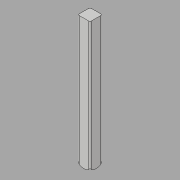
# Autodesk Inventor part: One_sided_axle_base-40_nogroove
Saved by Autodesk Inventor 2020 (Build 240168000, 168)
## iProperties
Created: 2018-11-05
Part Number: One_sided_axle_base-40_nogroove
Material: Generic
Description: Unknown
Document SubType Name: Modeling
Designer: Varga Daniel
Density: 1 g/cm^3
Appearance: Default
Company: Unknown
Sending System: DEX
Preprocessor: ST-DEVELOPER v16.7
Axle_length: 40,000 mm
Upper_fillet: 0,400 mm
Title: Axeis 2
Author: Unknown
Autodesk Inventor part; units mm, degrees
ref_plane "XZ Plane" through (0, 0, 0) normal (0, 1, 0) x (-1, 0, 0)
derived "Base_part.ipt"
sketch "Axle_sketch" plane through (0, 0, 0) normal (0, 1, 0) x (-1, 0, 0)
  circle A0 centre (0, 0) radius 2.5 construction
  line L0 (1.475, -1.875) -> (-1.475, -1.875)
  line L1 (-1.875, -1.475) -> (-1.875, 1.475)
  line L2 (-1.475, 1.875) -> (1.475, 1.875)
  line L3 (1.875, 1.475) -> (1.875, -1.475)
  line L4 (1.875, -1.875) -> (-1.875, 1.875) construction
  line L5 (-1.875, -1.875) -> (1.875, 1.875) construction
  arc A1 (1.475, -1.875) -> (1.875, -1.475) centre (1.475, -1.475) ccw
  arc A2 (-1.875, -1.475) -> (-1.475, -1.875) centre (-1.475, -1.475) ccw
  arc A3 (1.875, 1.475) -> (1.475, 1.875) centre (1.475, 1.475) ccw
  arc A4 (-1.475, 1.875) -> (-1.875, 1.475) centre (-1.475, 1.475) ccw
sketch "Sketch1" plane through (0, 0, 0) normal (0, 1, 0) x (-1, 0, 0)
  line L0 (-1.475, -1.875) -> (1.475, -1.875)
  line L1 (1.875, -1.475) -> (1.875, 1.475)
  line L2 (1.475, 1.875) -> (-1.475, 1.875)
  line L3 (-1.875, 1.475) -> (-1.875, -1.475)
  line L4 (-1.875, -1.875) -> (1.875, 1.875) construction
  line L5 (1.875, -1.875) -> (-1.875, 1.875) construction
  arc A0 (-1.875, -1.475) -> (-1.475, -1.875) centre (-1.475, -1.475) ccw
  arc A1 (1.475, -1.875) -> (1.875, -1.475) centre (1.475, -1.475) ccw
  arc A2 (1.875, 1.475) -> (1.475, 1.875) centre (1.475, 1.475) ccw
  arc A3 (-1.475, 1.875) -> (-1.875, 1.475) centre (-1.475, 1.475) ccw
  circle A4 centre (0, 0) radius 2.5 construction
  line L6 (1.475, -1.875) -> (-1.475, -1.875) construction
  arc A5 (1.475, -1.875) -> (1.875, -1.475) centre (1.475, -1.475) ccw construction
  line L7 (1.875, 1.475) -> (1.875, -1.475) construction
  circle A6 centre (0, 0) radius 2.5 construction
  line L8 (-1.475, 1.875) -> (1.475, 1.875) construction
  arc A7 (-1.475, 1.875) -> (-1.875, 1.475) centre (-1.475, 1.475) ccw construction
  line L9 (-1.875, -1.475) -> (-1.875, 1.475) construction
  arc A8 (-1.875, -1.475) -> (-1.475, -1.875) centre (-1.475, -1.475) ccw construction
  arc A9 (1.875, 1.475) -> (1.475, 1.875) centre (1.475, 1.475) ccw construction
  line L10 (-1.875, 1.875) -> (1.875, 1.875)
  line L11 (1.875, 1.875) -> (1.875, -1.875)
  line L12 (1.875, -1.875) -> (-1.875, -1.875)
  line L13 (-1.875, -1.875) -> (-1.875, 1.875)
  line L14 (1.875, -0.5) -> (0.875, -0.5)
  line L15 (0.875, -0.5) -> (0.875, 0.5)
  line L16 (0.875, 0.5) -> (1.875, 0.5)
  line L17 (1.875, 0.5) -> (1.875, -0.5)
  line L18 (-1.875, -0.5) -> (-0.875, -0.5)
  line L19 (-0.875, -0.5) -> (-0.875, 0.5)
  line L20 (-0.875, 0.5) -> (-1.875, 0.5)
  line L21 (-1.875, 0.5) -> (-1.875, -0.5)
  line L22 (-1.875, 0) -> (1.875, 0) construction
  point P0 (1.875, 1.475)
  point P1 (1.475, -1.875)
  point P2 (-1.875, -1.475)
  dimension "d0" = 3.75
  dimension "d1" = 3.75
  dimension "d2" = 0.4
  dimension "d11" = 5
  dimension "d13" = 3.75
  dimension "d14" = 0.4
  dimension "d31" = 1
  dimension "d32" = 1
  dimension "d33" = 1
  constraints: 38 end point, 12 point on line, 8 parallel, 8 point on circle, 8 tangent, 5 centre point, 5 midpoint, 4 collinear, 4 horizontal, 4 perpendicular, 3 equal radius, 1 coincident
  measures "d0" distance of L4.end L5.end
  measures "d1" distance between parallel lines of L2 L0
  measures "d2" radius of A0
  measures "d11" diameter of A4
  measures "d13" distance between parallel lines of L7 L9
  measures "d14" radius of A8
  measures "d31" distance between parallel lines of L16 L14
  measures "d32" distance between parallel lines of L11 L15
  measures "d33" distance between parallel lines of L9 L19
extrude "Extrusion4" add sketch "Sketch1" along normal blind 40
fillet "Fillet4" radius 0.4 4 edges at (-1.875, 20, 1.875) (1.875, 20, 1.875) (-1.875, 20, -1.875) (1.875, 20, -1.875)
ref_plane "Work Plane5" through (0, 0, 0) normal (-0.7071068, 0, 0.7071068) x (0, -1, 0)
extrude "Groove_extrusion" [suppressed]
sketch "Sketch8" plane through (1.875, 0, -1.475) normal (1, 0, 0) x (0, 0, -1)
  line L0 (-1.975, 20) -> (-0.975, 20) projected
  line L1 (-1.975, 0) -> (-1.975, 20) projected
  line L2 (-0.975, 0) -> (-1.975, 0) projected
  line L3 (-0.975, 0) -> (-0.975, 20) projected
  line L4 (-1.975, 0) -> (-0.975, 0)
  line L5 (-0.975, 0) -> (-0.975, 2)
  line L6 (-0.975, 2) -> (-1.975, 2)
  line L7 (-1.975, 2) -> (-1.975, 0)
  point P0 (-1.475, 0)
  dimension "d36" = 2
  constraints: 8 end point, 2 parallel, 1 horizontal, 1 perpendicular, 1 point on line
  measures "d36" distance between parallel lines of L6 L2
extrude "Extrusion6" [suppressed]
pattern_linear "Rectangular Pattern1" [suppressed]
sketch "Sketch7" plane through (0, 0, 0) normal (-0.7071068, 0, 0.7071068) x (0, -1, 0)
  line L0 (4.2485, 0) -> (-24.0414, 0) projected
  line L1 (0, 2.486) -> (0, -2.486) projected
  line L2 (0, -2.486) -> (-40, -2.486) projected
  line L3 (-40, -2.486) -> (-40, 2.486) projected
  line L4 (-40, 2.486) -> (0, 2.486) projected
  line L5 (0, 2.486) -> (-4, 2.486)
  line L6 (-4, 2.486) -> (-4, 0)
  line L7 (-4, 0) -> (0, 0)
  line L8 (0, 0) -> (0, 2.486)
  arc A0 (0, 1.486) -> (-1, 2.486) centre (-1, 1.486) ccw
  dimension "d29" = 4
  dimension "d30" = 1
  constraints: 8 end point, 3 point on line, 2 parallel, 2 point on circle, 2 tangent, 1 centre point, 1 horizontal, 1 perpendicular
  measures "d29" distance between parallel lines of L6 L8
  measures "d30" radius of A0
revolve "Revolution2" cut sketch "Sketch7" angle 360 about axis through (0, -10, 0) along (0, 1, 0) contours A0 L4 L1
equation "\"d0\" = d13"
equation "\"d1\" = d0"
equation "\"d2\" = d14"
equation "\"d31\" = Axle_groove_width"
equation "\"d32\" = Axle_groove_depth"
equation "\"d33\" = Axle_groove_depth"
equation "\"d15\" = Axle_length"
equation "\"d26\" = Axle_fillet"
equation "\"d30\" = Axle_end_fillet"
equation "\"Axle_length\" = 40"
equation "\"Upper_fillet\" = Axle_fillet"
equation "\"Axle_groove_width\" = 1"
equation "\"Axle_groove_depth\" = 1"
equation "\"Axle_fillet\" = 0.4"
equation "\"Axle_end_fillet\" = 1"
body "Solid1"
